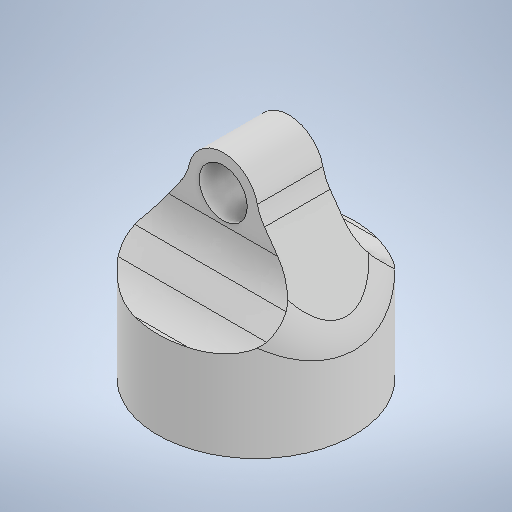
# Autodesk Inventor part: Odom_Part1
Saved by Autodesk Inventor 2025.1 (Build 291241020, 241B)
## iProperties
Created: 2024-09-26
Part Number: Odom_Part1
Material: Generic
Document SubType Name: Modeling
Designer: AtuStem
Density: 1 g/cm^3
Appearance: Default
Author: AtuStem
Autodesk Inventor part; units mm, degrees
ref_plane "YZ Plane" through (0, 0, 0) normal (1, 0, 0) x (0, 1, 0)
ref_plane "XZ Plane" through (0, 0, 0) normal (0, 1, 0) x (-1, 0, 0)
ref_plane "XY Plane" through (0, 0, 0) normal (0, 0, 1) x (1, 0, 0)
sketch "Sketch1" plane through (0, 0, 0) normal (0, 1, 0) x (-1, 0, 0)
  circle A0 centre (0, 0) radius 11.3665
  circle A1 centre (0, 0) radius 14.2875
  dimension "d0" = 22.733
  dimension "d1" = 28.575
  constraints: 2 centre point, 2 coincident
  measures "d0" diameter of A0
  measures "d1" diameter of A1
extrude "Extrusion1" add sketch "Sketch1" along normal blind 12.7
sketch "Sketch2" plane through (0, 12.7, 0) normal (0, 1, 0) x (1, 0, 0)
  circle A0 centre (0, 0) radius 14.2875 projected
  circle A1 centre (0, 0) radius 11.3665 projected
extrude "Extrusion2" add sketch "Sketch2" against normal blind 6.35 contours A1
sketch "Sketch3" plane through (0, 0, 0) normal (0, 0, 1) x (1, 0, 0)
  line L0 (14.2875, 12.7) -> (-14.2875, 12.7) projected
  line L1 (14.2875, 0) -> (-14.2875, 0) projected
  line L2 (0, 12.7) -> (0, 22.225)
  line L3 (0, 22.225) -> (0, 25.7175)
  circle A0 centre (0, 25.7175) radius 3.4925
  circle A1 centre (0, 25.7175) radius 5.08
  point P0 (0, 0)
  dimension "d6" = 9.525
  dimension "d7" = 3.4925
  dimension "d8" = 6.985
  dimension "d9" = 10.16
  constraints: 4 end point, 2 centre point, 2 coincident, 2 vertical, 1 midpoint
  measures "d6" distance of L2.start L2.end
  measures "d7" distance of L2.end L3.end
  measures "d8" diameter of A0
  measures "d9" diameter of A1
extrude "Extrusion3" add sketch "Sketch3" along normal mid plane 9.525
sketch "Sketch4" plane through (0, 25.7175, -4.7625) normal (0, 0, -1) x (-1, 0, 0)
  circle A0 centre (0, 0) radius 5.08 projected
  circle A1 centre (0, 0) radius 3.4925 projected
  line L0 (14.2875, -25.7175) -> (14.2875, -13.0175) projected
  line L1 (14.2875, -13.0175) -> (-14.2875, -13.0175) projected
  line L2 (14.2875, -25.7175) -> (-14.2875, -25.7175) projected
  line L3 (5.08, 0) -> (14.2875, -13.0175)
  line L4 (-5.08, 0) -> (-14.2875, -13.0175)
  line L5 (14.2875, -13.0175) -> (-14.2875, -13.0175) projected
  point P0 (0, -25.7175)
  constraints: 4 end point, 2 point on circle
extrude "Extrusion4" add sketch "Sketch4" against normal blind 9.525 contours L3 L1 L4 A0
sketch "Sketch5" plane through (-14.2875, 12.7, 4.7625) normal (0, -1, 0) x (1, 0, 0)
  circle A0 centre (14.2875, -4.7625) radius 14.2875 projected
  line L0 (28.575, -4.7625) -> (28.575, 0) projected
  arc A1 (28.575, -4.7625) -> (27.7579, 0) centre (14.2875, -4.7625) ccw projected
  line L1 (28.575, -4.7625) -> (28.575, 0) projected
  line L2 (27.7579, 0) -> (28.575, 0) projected
  arc A2 (27.7579, -9.525) -> (28.575, -4.7625) centre (14.2875, -4.7625) ccw projected
  line L3 (28.575, -9.525) -> (27.7579, -9.525) projected
  line L4 (28.575, -9.525) -> (28.575, -4.7625) projected
  arc A3 (0.8171, 0) -> (0, -4.7625) centre (14.2875, -4.7625) ccw projected
  line L5 (0, 0) -> (0.8171, 0) projected
  line L6 (0, -4.7625) -> (0, 0) projected
  arc A4 (0, -4.7625) -> (0.8171, -9.525) centre (14.2875, -4.7625) ccw projected
  line L7 (0, -9.525) -> (0, -4.7625) projected
  line L8 (0.8171, -9.525) -> (0, -9.525) projected
  circle A5 centre (14.2875, -4.7625) radius 14.2875 projected
  circle A6 centre (14.2875, -4.7625) radius 11.3665 projected
  point P0 (27.7579, 0)
  point P1 (27.7579, -9.525)
  point P2 (0.8171, -9.525)
  point P3 (0, -4.7625)
  point P4 (0, -4.7625)
  point P5 (0, -4.7625)
  point P6 (0.8171, 0)
  constraints: 1 other
extrude "Extrusion5" cut sketch "Sketch5" against normal blind 9.525 contours L4 L3 A0 | A0 L2 L0 | A0 L6 L5 | L8 L7 A0
chamfer "Chamfer1" distance 6.35 angle 45 1 edges at (0, 12.7, 4.7625)
chamfer "Chamfer2" distance 6.35 angle 45 1 edges at (0, 12.7, -4.7625)
fillet "Fillet1" radius 6.35 14 edges at (0, 12.7, 11.1125) (0, 19.05, 4.7625) (0, 19.05, -4.7625) (0, 12.7, -11.1125) (12.8057, 14.7949, 6.3361) (14.0817, 12.9909, 2.416) (12.8057, 14.7949, -6.3361) (14.0817, 12.9909, -2.416) (-14.0817, 12.9909, -2.416) (-14.0817, 12.9909, 2.416) (-12.8057, 14.7949, 6.3361) (-12.8057, 14.7949, -6.3361) (5.08, 25.7175, 0) (-5.08, 25.7175, 0)
body "Solid1"
